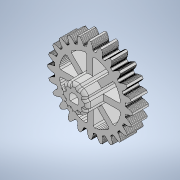
# Autodesk Inventor part: Ведущая шестерня дифференециала 24
Saved by Autodesk Inventor 2020 (Build 240168000, 168)
## iProperties
Created: 2021-10-09
Part Number: Ведущая шестерня дифференециала 24
Material: Типовые
Document SubType Name: Modeling
Designer: Антон
Density: 1 g/cm^3
Appearance: По умолчанию
Autodesk Inventor part; units mm, degrees
ref_plane "YZ Plane" through (0, 0, 0) normal (1, 0, 0) x (0, 1, 0)
ref_plane "XZ Plane" through (0, 0, 0) normal (0, 1, 0) x (-1, 0, 0)
ref_plane "XY Plane" through (0, 0, 0) normal (0, 0, 1) x (1, 0, 0)
sketch "a" plane through (0, 0, 0) normal (0, 0, 1) x (1, 0, 0)
  line L0 (2.2314, 12.0308) -> (2.1649, 12.1461)
  line L1 (2.1649, 12.1461) -> (2.1066, 12.1863)
  line L2 (2.1066, 12.1863) -> (2.0498, 12.2129)
  line L3 (2.0498, 12.2129) -> (1.9381, 12.246)
  line L4 (1.9381, 12.246) -> (1.8277, 12.2671)
  line L5 (1.8277, 12.2671) -> (1.7187, 12.2707)
  line L6 (1.7187, 12.2707) -> (1.4993, 12.2976)
  line L7 (1.4993, 12.2976) -> (1.2787, 12.3426)
  line L8 (1.2787, 12.3426) -> (1.0573, 12.4024)
  line L9 (1.0573, 12.4024) -> (0.8356, 12.4754)
  line L10 (0.8356, 12.4754) -> (0.6138, 12.5604)
  line L11 (0.6138, 12.5604) -> (0.3923, 12.6568)
  line L12 (0.3923, 12.6568) -> (0.1712, 12.7641)
  line L13 (0.1712, 12.7641) -> (0.0059, 12.8514)
  line L14 (0.0059, 12.8514) -> (0.0025, 13.5004)
  line L15 (0.0025, 13.5004) -> (0.1669, 13.5895)
  line L16 (0.1669, 13.5895) -> (0.3868, 13.699)
  line L17 (0.3868, 13.699) -> (0.6073, 13.7977)
  line L18 (0.6073, 13.7977) -> (0.8282, 13.8851)
  line L19 (0.8282, 13.8851) -> (1.0492, 13.9604)
  line L20 (1.0492, 13.9604) -> (1.2699, 14.0225)
  line L21 (1.2699, 14.0225) -> (1.49, 14.0699)
  line L22 (1.49, 14.0699) -> (1.7092, 14.099)
  line L23 (1.7092, 14.099) -> (1.818, 14.1038)
  line L24 (1.818, 14.1038) -> (1.9283, 14.126)
  line L25 (1.9283, 14.126) -> (2.0396, 14.1603)
  line L26 (2.0396, 14.1603) -> (2.0962, 14.1875)
  line L27 (2.0962, 14.1875) -> (2.154, 14.2283)
  line L28 (2.154, 14.2283) -> (2.2193, 14.3443)
  line L29 (2.2193, 14.3443) -> (2.2924, 14.9228)
  line L30 (2.2924, 14.9228) -> (2.258, 15.0513)
  line L31 (2.258, 15.0513) -> (2.2121, 15.1053)
  line L32 (2.2121, 15.1053) -> (2.1641, 15.1457)
  line L33 (2.1641, 15.1457) -> (2.0648, 15.2066)
  line L34 (2.0648, 15.2066) -> (1.9635, 15.2555)
  line L35 (1.9635, 15.2555) -> (1.8593, 15.2872)
  line L36 (1.8593, 15.2872) -> (1.6543, 15.3699)
  line L37 (1.6543, 15.3699) -> (1.4528, 15.4705)
  line L38 (1.4528, 15.4705) -> (1.2545, 15.5856)
  line L39 (1.2545, 15.5856) -> (1.0592, 15.7135)
  line L40 (1.0592, 15.7135) -> (0.867, 15.853)
  line L41 (0.867, 15.853) -> (0.6779, 16.0035)
  line L42 (0.6779, 16.0035) -> (0.4922, 16.1643)
  line L43 (0.4922, 16.1643) -> (0.355, 16.2914)
  line L44 (0.355, 16.2914) -> (0.5198, 16.9192)
  line L45 (0.5198, 16.9192) -> (0.7016, 16.9627)
  line L46 (0.7016, 16.9627) -> (0.9424, 17.0116)
  line L47 (0.9424, 17.0116) -> (1.181, 17.0498)
  line L48 (1.181, 17.0498) -> (1.4169, 17.077)
  line L49 (1.4169, 17.077) -> (1.6498, 17.0926)
  line L50 (1.6498, 17.0926) -> (1.8791, 17.0955)
  line L51 (1.8791, 17.0955) -> (2.104, 17.0842)
  line L52 (2.104, 17.0842) -> (2.3232, 17.0556)
  line L53 (2.3232, 17.0556) -> (2.4296, 17.0321)
  line L54 (2.4296, 17.0321) -> (2.5419, 17.025)
  line L55 (2.5419, 17.025) -> (2.6582, 17.0293)
  line L56 (2.6582, 17.0293) -> (2.7199, 17.041)
  line L57 (2.7199, 17.041) -> (2.7864, 17.0654)
  line L58 (2.7864, 17.0654) -> (2.8795, 17.1606)
  line L59 (2.8795, 17.1606) -> (3.0998, 17.7004)
  line L60 (3.0998, 17.7004) -> (3.0998, 17.8335)
  line L61 (3.0998, 17.8335) -> (3.0695, 17.8975)
  line L62 (3.0695, 17.8975) -> (3.0335, 17.9489)
  line L63 (3.0335, 17.9489) -> (2.9534, 18.0335)
  line L64 (2.9534, 18.0335) -> (2.8682, 18.1069)
  line L65 (2.8682, 18.1069) -> (2.7757, 18.1646)
  line L66 (2.7757, 18.1646) -> (2.5991, 18.2975)
  line L67 (2.5991, 18.2975) -> (2.4306, 18.4468)
  line L68 (2.4306, 18.4468) -> (2.2688, 18.6093)
  line L69 (2.2688, 18.6093) -> (2.1133, 18.7833)
  line L70 (2.1133, 18.7833) -> (1.9637, 18.9679)
  line L71 (1.9637, 18.9679) -> (1.82, 19.1621)
  line L72 (1.82, 19.1621) -> (1.6822, 19.3655)
  line L73 (1.6822, 19.3655) -> (1.5827, 19.5238)
  line L74 (1.5827, 19.5238) -> (1.9043, 20.0876)
  line L75 (1.9043, 20.0876) -> (2.0912, 20.0825)
  line L76 (2.0912, 20.0825) -> (2.3364, 20.0674)
  line L77 (2.3364, 20.0674) -> (2.5768, 20.0427)
  line L78 (2.5768, 20.0427) -> (2.8117, 20.0079)
  line L79 (2.8117, 20.0079) -> (3.0407, 19.9626)
  line L80 (3.0407, 19.9626) -> (3.2629, 19.9061)
  line L81 (3.2629, 19.9061) -> (3.4772, 19.837)
  line L82 (3.4772, 19.837) -> (3.6816, 19.7526)
  line L83 (3.6816, 19.7526) -> (3.7783, 19.7024)
  line L84 (3.7783, 19.7024) -> (3.8848, 19.6665)
  line L85 (3.8848, 19.6665) -> (3.9984, 19.6405)
  line L86 (3.9984, 19.6405) -> (4.061, 19.6358)
  line L87 (4.061, 19.6358) -> (4.1315, 19.6422)
  line L88 (4.1315, 19.6422) -> (4.246, 19.71)
  line L89 (4.246, 19.71) -> (4.5985, 20.1744)
  line L90 (4.5985, 20.1744) -> (4.633, 20.303)
  line L91 (4.633, 20.303) -> (4.6203, 20.3726)
  line L92 (4.6203, 20.3726) -> (4.5989, 20.4317)
  line L93 (4.5989, 20.4317) -> (4.5434, 20.534)
  line L94 (4.5434, 20.534) -> (4.4801, 20.627)
  line L95 (4.4801, 20.627) -> (4.4057, 20.7066)
  line L96 (4.4057, 20.7066) -> (4.2695, 20.8808)
  line L97 (4.2695, 20.8808) -> (4.1453, 21.0686)
  line L98 (4.1453, 21.0686) -> (4.0311, 21.2675)
  line L99 (4.0311, 21.2675) -> (3.9259, 21.4758)
  line L100 (3.9259, 21.4758) -> (3.8292, 21.6928)
  line L101 (3.8292, 21.6928) -> (3.7407, 21.9176)
  line L102 (3.7407, 21.9176) -> (3.6603, 22.1497)
  line L103 (3.6603, 22.1497) -> (3.6051, 22.3284)
  line L104 (3.6051, 22.3284) -> (4.0616, 22.7898)
  line L105 (4.0616, 22.7898) -> (4.2409, 22.7365)
  line L106 (4.2409, 22.7365) -> (4.4738, 22.6584)
  line L107 (4.4738, 22.6584) -> (4.6996, 22.5723)
  line L108 (4.6996, 22.5723) -> (4.9175, 22.4778)
  line L109 (4.9175, 22.4778) -> (5.127, 22.3748)
  line L110 (5.127, 22.3748) -> (5.327, 22.2627)
  line L111 (5.327, 22.2627) -> (5.5161, 22.1405)
  line L112 (5.5161, 22.1405) -> (5.6917, 22.0062)
  line L113 (5.6917, 22.0062) -> (5.7721, 21.9326)
  line L114 (5.7721, 21.9326) -> (5.8657, 21.8703)
  line L115 (5.8657, 21.8703) -> (5.9687, 21.8158)
  line L116 (5.9687, 21.8158) -> (6.0279, 21.7951)
  line L117 (6.0279, 21.7951) -> (6.0977, 21.783)
  line L118 (6.0977, 21.783) -> (6.2259, 21.8189)
  line L119 (6.2259, 21.8189) -> (6.6866, 22.1763)
  line L120 (6.6866, 22.1763) -> (6.7532, 22.2915)
  line L121 (6.7532, 22.2915) -> (6.7589, 22.3621)
  line L122 (6.7589, 22.3621) -> (6.7535, 22.4246)
  line L123 (6.7535, 22.4246) -> (6.7264, 22.5379)
  line L124 (6.7264, 22.5379) -> (6.6893, 22.6441)
  line L125 (6.6893, 22.6441) -> (6.638, 22.7402)
  line L126 (6.638, 22.7402) -> (6.5516, 22.9437)
  line L127 (6.5516, 22.9437) -> (6.4803, 23.1573)
  line L128 (6.4803, 23.1573) -> (6.4214, 23.3789)
  line L129 (6.4214, 23.3789) -> (6.3737, 23.6074)
  line L130 (6.3737, 23.6074) -> (6.3365, 23.842)
  line L131 (6.3365, 23.842) -> (6.3092, 24.082)
  line L132 (6.3092, 24.082) -> (6.2915, 24.3271)
  line L133 (6.2915, 24.3271) -> (6.2845, 24.5139)
  line L134 (6.2845, 24.5139) -> (6.8449, 24.8414)
  line L135 (6.8449, 24.8414) -> (7.0042, 24.7435)
  line L136 (7.0042, 24.7435) -> (7.209, 24.6078)
  line L137 (7.209, 24.6078) -> (7.4048, 24.4662)
  line L138 (7.4048, 24.4662) -> (7.5908, 24.3186)
  line L139 (7.5908, 24.3186) -> (7.7665, 24.1649)
  line L140 (7.7665, 24.1649) -> (7.9307, 24.0048)
  line L141 (7.9307, 24.0048) -> (8.0818, 23.8378)
  line L142 (8.0818, 23.8378) -> (8.2165, 23.6626)
  line L143 (8.2165, 23.6626) -> (8.2752, 23.5708)
  line L144 (8.2752, 23.5708) -> (8.3495, 23.4864)
  line L145 (8.3495, 23.4864) -> (8.4348, 23.4071)
  line L146 (8.4348, 23.4071) -> (8.4867, 23.3717)
  line L147 (8.4867, 23.3717) -> (8.551, 23.342)
  line L148 (8.551, 23.342) -> (8.6841, 23.3435)
  line L149 (8.6841, 23.3435) -> (9.2216, 23.5695)
  line L150 (9.2216, 23.5695) -> (9.3157, 23.6635)
  line L151 (9.3157, 23.6635) -> (9.3395, 23.7302)
  line L152 (9.3395, 23.7302) -> (9.3505, 23.792)
  line L153 (9.3505, 23.792) -> (9.3536, 23.9085)
  line L154 (9.3536, 23.9085) -> (9.3453, 24.0206)
  line L155 (9.3453, 24.0206) -> (9.3207, 24.1268)
  line L156 (9.3207, 24.1268) -> (9.2898, 24.3457)
  line L157 (9.2898, 24.3457) -> (9.2762, 24.5704)
  line L158 (9.2762, 24.5704) -> (9.2767, 24.7997)
  line L159 (9.2767, 24.7997) -> (9.2898, 25.0328)
  line L160 (9.2898, 25.0328) -> (9.3145, 25.269)
  line L161 (9.3145, 25.269) -> (9.3503, 25.508)
  line L162 (9.3503, 25.508) -> (9.3966, 25.7493)
  line L163 (9.3966, 25.7493) -> (9.4382, 25.9316)
  line L164 (9.4382, 25.9316) -> (10.0643, 26.1028)
  line L165 (10.0643, 26.1028) -> (10.1928, 25.9671)
  line L166 (10.1928, 25.9671) -> (10.3556, 25.783)
  line L167 (10.3556, 25.783) -> (10.508, 25.5955)
  line L168 (10.508, 25.5955) -> (10.6495, 25.4048)
  line L169 (10.6495, 25.4048) -> (10.7794, 25.2108)
  line L170 (10.7794, 25.2108) -> (10.8966, 25.0137)
  line L171 (10.8966, 25.0137) -> (10.9993, 24.8133)
  line L172 (10.9993, 24.8133) -> (11.0841, 24.6092)
  line L173 (11.0841, 24.6092) -> (11.117, 24.5053)
  line L174 (11.117, 24.5053) -> (11.1669, 24.4045)
  line L175 (11.1669, 24.4045) -> (11.2288, 24.3059)
  line L176 (11.2288, 24.3059) -> (11.2698, 24.2583)
  line L177 (11.2698, 24.2583) -> (11.3242, 24.213)
  line L178 (11.3242, 24.213) -> (11.4531, 24.1799)
  line L179 (11.4531, 24.1799) -> (12.0308, 24.2591)
  line L180 (12.0308, 24.2591) -> (12.1461, 24.3256)
  line L181 (12.1461, 24.3256) -> (12.1863, 24.3838)
  line L182 (12.1863, 24.3838) -> (12.2129, 24.4407)
  line L183 (12.2129, 24.4407) -> (12.246, 24.5523)
  line L184 (12.246, 24.5523) -> (12.2671, 24.6628)
  line L185 (12.2671, 24.6628) -> (12.2707, 24.7718)
  line L186 (12.2707, 24.7718) -> (12.2976, 24.9912)
  line L187 (12.2976, 24.9912) -> (12.3426, 25.2118)
  line L188 (12.3426, 25.2118) -> (12.4024, 25.4332)
  line L189 (12.4024, 25.4332) -> (12.4754, 25.6549)
  line L190 (12.4754, 25.6549) -> (12.5604, 25.8766)
  line L191 (12.5604, 25.8766) -> (12.6568, 26.0982)
  line L192 (12.6568, 26.0982) -> (12.7641, 26.3193)
  line L193 (12.7641, 26.3193) -> (12.8514, 26.4846)
  line L194 (12.8514, 26.4846) -> (13.5004, 26.488)
  line L195 (13.5004, 26.488) -> (13.5895, 26.3236)
  line L196 (13.5895, 26.3236) -> (13.699, 26.1036)
  line L197 (13.699, 26.1036) -> (13.7977, 25.8831)
  line L198 (13.7977, 25.8831) -> (13.8851, 25.6623)
  line L199 (13.8851, 25.6623) -> (13.9604, 25.4413)
  line L200 (13.9604, 25.4413) -> (14.0225, 25.2206)
  line L201 (14.0225, 25.2206) -> (14.0699, 25.0005)
  line L202 (14.0699, 25.0005) -> (14.099, 24.7813)
  line L203 (14.099, 24.7813) -> (14.1038, 24.6724)
  line L204 (14.1038, 24.6724) -> (14.126, 24.5622)
  line L205 (14.126, 24.5622) -> (14.1603, 24.4509)
  line L206 (14.1603, 24.4509) -> (14.1875, 24.3943)
  line L207 (14.1875, 24.3943) -> (14.2283, 24.3365)
  line L208 (14.2283, 24.3365) -> (14.3443, 24.2712)
  line L209 (14.3443, 24.2712) -> (14.9228, 24.1981)
  line L210 (14.9228, 24.1981) -> (15.0513, 24.2325)
  line L211 (15.0513, 24.2325) -> (15.1053, 24.2784)
  line L212 (15.1053, 24.2784) -> (15.1457, 24.3264)
  line L213 (15.1457, 24.3264) -> (15.2066, 24.4257)
  line L214 (15.2066, 24.4257) -> (15.2555, 24.5269)
  line L215 (15.2555, 24.5269) -> (15.2872, 24.6312)
  line L216 (15.2872, 24.6312) -> (15.3699, 24.8362)
  line L217 (15.3699, 24.8362) -> (15.4705, 25.0377)
  line L218 (15.4705, 25.0377) -> (15.5856, 25.236)
  line L219 (15.5856, 25.236) -> (15.7135, 25.4313)
  line L220 (15.7135, 25.4313) -> (15.853, 25.6235)
  line L221 (15.853, 25.6235) -> (16.0035, 25.8125)
  line L222 (16.0035, 25.8125) -> (16.1643, 25.9983)
  line L223 (16.1643, 25.9983) -> (16.2914, 26.1354)
  line L224 (16.2914, 26.1354) -> (16.9192, 25.9707)
  line L225 (16.9192, 25.9707) -> (16.9627, 25.7889)
  line L226 (16.9627, 25.7889) -> (17.0116, 25.5481)
  line L227 (17.0116, 25.5481) -> (17.0498, 25.3095)
  line L228 (17.0498, 25.3095) -> (17.077, 25.0736)
  line L229 (17.077, 25.0736) -> (17.0926, 24.8407)
  line L230 (17.0926, 24.8407) -> (17.0955, 24.6114)
  line L231 (17.0955, 24.6114) -> (17.0842, 24.3865)
  line L232 (17.0842, 24.3865) -> (17.0556, 24.1673)
  line L233 (17.0556, 24.1673) -> (17.0321, 24.0609)
  line L234 (17.0321, 24.0609) -> (17.025, 23.9486)
  line L235 (17.025, 23.9486) -> (17.0293, 23.8322)
  line L236 (17.0293, 23.8322) -> (17.041, 23.7705)
  line L237 (17.041, 23.7705) -> (17.0654, 23.7041)
  line L238 (17.0654, 23.7041) -> (17.1606, 23.611)
  line L239 (17.1606, 23.611) -> (17.7004, 23.3907)
  line L240 (17.7004, 23.3907) -> (17.8335, 23.3907)
  line L241 (17.8335, 23.3907) -> (17.8975, 23.421)
  line L242 (17.8975, 23.421) -> (17.9489, 23.4569)
  line L243 (17.9489, 23.4569) -> (18.0335, 23.5371)
  line L244 (18.0335, 23.5371) -> (18.1069, 23.6222)
  line L245 (18.1069, 23.6222) -> (18.1646, 23.7147)
  line L246 (18.1646, 23.7147) -> (18.2975, 23.8913)
  line L247 (18.2975, 23.8913) -> (18.4468, 24.0599)
  line L248 (18.4468, 24.0599) -> (18.6093, 24.2217)
  line L249 (18.6093, 24.2217) -> (18.7833, 24.3772)
  line L250 (18.7833, 24.3772) -> (18.9679, 24.5268)
  line L251 (18.9679, 24.5268) -> (19.1621, 24.6704)
  line L252 (19.1621, 24.6704) -> (19.3655, 24.8083)
  line L253 (19.3655, 24.8083) -> (19.5238, 24.9078)
  line L254 (19.5238, 24.9078) -> (20.0876, 24.5862)
  line L255 (20.0876, 24.5862) -> (20.0825, 24.3993)
  line L256 (20.0825, 24.3993) -> (20.0674, 24.1541)
  line L257 (20.0674, 24.1541) -> (20.0427, 23.9137)
  line L258 (20.0427, 23.9137) -> (20.0079, 23.6788)
  line L259 (20.0079, 23.6788) -> (19.9626, 23.4498)
  line L260 (19.9626, 23.4498) -> (19.9061, 23.2276)
  line L261 (19.9061, 23.2276) -> (19.837, 23.0132)
  line L262 (19.837, 23.0132) -> (19.7526, 22.8089)
  line L263 (19.7526, 22.8089) -> (19.7024, 22.7122)
  line L264 (19.7024, 22.7122) -> (19.6665, 22.6056)
  line L265 (19.6665, 22.6056) -> (19.6405, 22.4921)
  line L266 (19.6405, 22.4921) -> (19.6358, 22.4295)
  line L267 (19.6358, 22.4295) -> (19.6422, 22.359)
  line L268 (19.6422, 22.359) -> (19.71, 22.2445)
  line L269 (19.71, 22.2445) -> (20.1744, 21.8919)
  line L270 (20.1744, 21.8919) -> (20.303, 21.8574)
  line L271 (20.303, 21.8574) -> (20.3726, 21.8702)
  line L272 (20.3726, 21.8702) -> (20.4317, 21.8916)
  line L273 (20.4317, 21.8916) -> (20.534, 21.9471)
  line L274 (20.534, 21.9471) -> (20.627, 22.0104)
  line L275 (20.627, 22.0104) -> (20.7066, 22.0848)
  line L276 (20.7066, 22.0848) -> (20.8808, 22.221)
  line L277 (20.8808, 22.221) -> (21.0686, 22.3451)
  line L278 (21.0686, 22.3451) -> (21.2675, 22.4593)
  line L279 (21.2675, 22.4593) -> (21.4758, 22.5645)
  line L280 (21.4758, 22.5645) -> (21.6928, 22.6612)
  line L281 (21.6928, 22.6612) -> (21.9176, 22.7497)
  line L282 (21.9176, 22.7497) -> (22.1497, 22.8302)
  line L283 (22.1497, 22.8302) -> (22.3284, 22.8854)
  line L284 (22.3284, 22.8854) -> (22.7898, 22.4288)
  line L285 (22.7898, 22.4288) -> (22.7365, 22.2496)
  line L286 (22.7365, 22.2496) -> (22.6584, 22.0166)
  line L287 (22.6584, 22.0166) -> (22.5723, 21.7909)
  line L288 (22.5723, 21.7909) -> (22.4778, 21.5729)
  line L289 (22.4778, 21.5729) -> (22.3748, 21.3635)
  line L290 (22.3748, 21.3635) -> (22.2627, 21.1635)
  line L291 (22.2627, 21.1635) -> (22.1405, 20.9743)
  line L292 (22.1405, 20.9743) -> (22.0062, 20.7988)
  line L293 (22.0062, 20.7988) -> (21.9326, 20.7184)
  line L294 (21.9326, 20.7184) -> (21.8703, 20.6247)
  line L295 (21.8703, 20.6247) -> (21.8158, 20.5218)
  line L296 (21.8158, 20.5218) -> (21.7951, 20.4626)
  line L297 (21.7951, 20.4626) -> (21.783, 20.3928)
  line L298 (21.783, 20.3928) -> (21.8189, 20.2646)
  line L299 (21.8189, 20.2646) -> (22.1763, 19.8039)
  line L300 (22.1763, 19.8039) -> (22.2915, 19.7373)
  line L301 (22.2915, 19.7373) -> (22.3621, 19.7316)
  line L302 (22.3621, 19.7316) -> (22.4246, 19.737)
  line L303 (22.4246, 19.737) -> (22.5379, 19.7641)
  line L304 (22.5379, 19.7641) -> (22.6441, 19.8011)
  line L305 (22.6441, 19.8011) -> (22.7402, 19.8524)
  line L306 (22.7402, 19.8524) -> (22.9437, 19.9389)
  line L307 (22.9437, 19.9389) -> (23.1573, 20.0102)
  line L308 (23.1573, 20.0102) -> (23.3789, 20.0691)
  line L309 (23.3789, 20.0691) -> (23.6074, 20.1167)
  line L310 (23.6074, 20.1167) -> (23.842, 20.154)
  line L311 (23.842, 20.154) -> (24.082, 20.1813)
  line L312 (24.082, 20.1813) -> (24.3271, 20.199)
  line L313 (24.3271, 20.199) -> (24.5139, 20.206)
  line L314 (24.5139, 20.206) -> (24.8414, 19.6456)
  line L315 (24.8414, 19.6456) -> (24.7435, 19.4863)
  line L316 (24.7435, 19.4863) -> (24.6078, 19.2814)
  line L317 (24.6078, 19.2814) -> (24.4662, 19.0857)
  line L318 (24.4662, 19.0857) -> (24.3186, 18.8996)
  line L319 (24.3186, 18.8996) -> (24.1649, 18.724)
  line L320 (24.1649, 18.724) -> (24.0048, 18.5598)
  line L321 (24.0048, 18.5598) -> (23.8378, 18.4087)
  line L322 (23.8378, 18.4087) -> (23.6626, 18.2739)
  line L323 (23.6626, 18.2739) -> (23.5708, 18.2153)
  line L324 (23.5708, 18.2153) -> (23.4864, 18.141)
  line L325 (23.4864, 18.141) -> (23.4071, 18.0556)
  line L326 (23.4071, 18.0556) -> (23.3717, 18.0038)
  line L327 (23.3717, 18.0038) -> (23.342, 17.9395)
  line L328 (23.342, 17.9395) -> (23.3435, 17.8064)
  line L329 (23.3435, 17.8064) -> (23.5695, 17.2689)
  line L330 (23.5695, 17.2689) -> (23.6635, 17.1747)
  line L331 (23.6635, 17.1747) -> (23.7302, 17.151)
  line L332 (23.7302, 17.151) -> (23.792, 17.14)
  line L333 (23.792, 17.14) -> (23.9085, 17.1369)
  line L334 (23.9085, 17.1369) -> (24.0206, 17.1452)
  line L335 (24.0206, 17.1452) -> (24.1268, 17.1698)
  line L336 (24.1268, 17.1698) -> (24.3457, 17.2007)
  line L337 (24.3457, 17.2007) -> (24.5704, 17.2143)
  line L338 (24.5704, 17.2143) -> (24.7997, 17.2138)
  line L339 (24.7997, 17.2138) -> (25.0328, 17.2007)
  line L340 (25.0328, 17.2007) -> (25.269, 17.176)
  line L341 (25.269, 17.176) -> (25.508, 17.1402)
  line L342 (25.508, 17.1402) -> (25.7493, 17.0938)
  line L343 (25.7493, 17.0938) -> (25.9316, 17.0523)
  line L344 (25.9316, 17.0523) -> (26.1028, 16.4262)
  line L345 (26.1028, 16.4262) -> (25.9671, 16.2977)
  line L346 (25.9671, 16.2977) -> (25.783, 16.1349)
  line L347 (25.783, 16.1349) -> (25.5955, 15.9825)
  line L348 (25.5955, 15.9825) -> (25.4048, 15.8409)
  line L349 (25.4048, 15.8409) -> (25.2108, 15.7111)
  line L350 (25.2108, 15.7111) -> (25.0137, 15.5939)
  line L351 (25.0137, 15.5939) -> (24.8133, 15.4912)
  line L352 (24.8133, 15.4912) -> (24.6092, 15.4063)
  line L353 (24.6092, 15.4063) -> (24.5053, 15.3735)
  line L354 (24.5053, 15.3735) -> (24.4045, 15.3235)
  line L355 (24.4045, 15.3235) -> (24.3059, 15.2616)
  line L356 (24.3059, 15.2616) -> (24.2583, 15.2207)
  line L357 (24.2583, 15.2207) -> (24.213, 15.1663)
  line L358 (24.213, 15.1663) -> (24.1799, 15.0374)
  line L359 (24.1799, 15.0374) -> (24.2591, 14.4597)
  line L360 (24.2591, 14.4597) -> (24.3256, 14.3444)
  line L361 (24.3256, 14.3444) -> (24.3838, 14.3042)
  line L362 (24.3838, 14.3042) -> (24.4407, 14.2776)
  line L363 (24.4407, 14.2776) -> (24.5523, 14.2444)
  line L364 (24.5523, 14.2444) -> (24.6628, 14.2234)
  line L365 (24.6628, 14.2234) -> (24.7718, 14.2197)
  line L366 (24.7718, 14.2197) -> (24.9912, 14.1929)
  line L367 (24.9912, 14.1929) -> (25.2118, 14.1479)
  line L368 (25.2118, 14.1479) -> (25.4332, 14.088)
  line L369 (25.4332, 14.088) -> (25.6549, 14.0151)
  line L370 (25.6549, 14.0151) -> (25.8766, 13.9301)
  line L371 (25.8766, 13.9301) -> (26.0982, 13.8337)
  line L372 (26.0982, 13.8337) -> (26.3193, 13.7264)
  line L373 (26.3193, 13.7264) -> (26.4846, 13.6391)
  line L374 (26.4846, 13.6391) -> (26.488, 12.99)
  line L375 (26.488, 12.99) -> (26.3236, 12.901)
  line L376 (26.3236, 12.901) -> (26.1036, 12.7914)
  line L377 (26.1036, 12.7914) -> (25.8831, 12.6927)
  line L378 (25.8831, 12.6927) -> (25.6623, 12.6054)
  line L379 (25.6623, 12.6054) -> (25.4413, 12.5301)
  line L380 (25.4413, 12.5301) -> (25.2206, 12.468)
  line L381 (25.2206, 12.468) -> (25.0005, 12.4206)
  line L382 (25.0005, 12.4206) -> (24.7813, 12.3915)
  line L383 (24.7813, 12.3915) -> (24.6724, 12.3867)
  line L384 (24.6724, 12.3867) -> (24.5622, 12.3645)
  line L385 (24.5622, 12.3645) -> (24.4509, 12.3302)
  line L386 (24.4509, 12.3302) -> (24.3943, 12.303)
  line L387 (24.3943, 12.303) -> (24.3365, 12.2622)
  line L388 (24.3365, 12.2622) -> (24.2712, 12.1462)
  line L389 (24.2712, 12.1462) -> (24.1981, 11.5677)
  line L390 (24.1981, 11.5677) -> (24.2325, 11.4391)
  line L391 (24.2325, 11.4391) -> (24.2784, 11.3852)
  line L392 (24.2784, 11.3852) -> (24.3264, 11.3448)
  line L393 (24.3264, 11.3448) -> (24.4257, 11.2839)
  line L394 (24.4257, 11.2839) -> (24.5269, 11.235)
  line L395 (24.5269, 11.235) -> (24.6312, 11.2032)
  line L396 (24.6312, 11.2032) -> (24.8362, 11.1205)
  line L397 (24.8362, 11.1205) -> (25.0377, 11.0199)
  line L398 (25.0377, 11.0199) -> (25.236, 10.9048)
  line L399 (25.236, 10.9048) -> (25.4313, 10.777)
  line L400 (25.4313, 10.777) -> (25.6235, 10.6375)
  line L401 (25.6235, 10.6375) -> (25.8125, 10.487)
  line L402 (25.8125, 10.487) -> (25.9983, 10.3262)
  line L403 (25.9983, 10.3262) -> (26.1354, 10.1991)
  line L404 (26.1354, 10.1991) -> (25.9707, 9.5712)
  line L405 (25.9707, 9.5712) -> (25.7889, 9.5278)
  line L406 (25.7889, 9.5278) -> (25.5481, 9.4789)
  line L407 (25.5481, 9.4789) -> (25.3095, 9.4406)
  line L408 (25.3095, 9.4406) -> (25.0736, 9.4134)
  line L409 (25.0736, 9.4134) -> (24.8407, 9.3979)
  line L410 (24.8407, 9.3979) -> (24.6114, 9.395)
  line L411 (24.6114, 9.395) -> (24.3865, 9.4062)
  line L412 (24.3865, 9.4062) -> (24.1673, 9.4348)
  line L413 (24.1673, 9.4348) -> (24.0609, 9.4584)
  line L414 (24.0609, 9.4584) -> (23.9486, 9.4655)
  line L415 (23.9486, 9.4655) -> (23.8322, 9.4612)
  line L416 (23.8322, 9.4612) -> (23.7705, 9.4495)
  line L417 (23.7705, 9.4495) -> (23.7041, 9.4251)
  line L418 (23.7041, 9.4251) -> (23.611, 9.3299)
  line L419 (23.611, 9.3299) -> (23.3907, 8.7901)
  line L420 (23.3907, 8.7901) -> (23.3907, 8.657)
  line L421 (23.3907, 8.657) -> (23.421, 8.593)
  line L422 (23.421, 8.593) -> (23.4569, 8.5415)
  line L423 (23.4569, 8.5415) -> (23.5371, 8.457)
  line L424 (23.5371, 8.457) -> (23.6222, 8.3836)
  line L425 (23.6222, 8.3836) -> (23.7147, 8.3259)
  line L426 (23.7147, 8.3259) -> (23.8913, 8.193)
  line L427 (23.8913, 8.193) -> (24.0599, 8.0436)
  line L428 (24.0599, 8.0436) -> (24.2217, 7.8811)
  line L429 (24.2217, 7.8811) -> (24.3772, 7.7071)
  line L430 (24.3772, 7.7071) -> (24.5268, 7.5226)
  line L431 (24.5268, 7.5226) -> (24.6704, 7.3283)
  line L432 (24.6704, 7.3283) -> (24.8083, 7.1249)
  line L433 (24.8083, 7.1249) -> (24.9078, 6.9666)
  line L434 (24.9078, 6.9666) -> (24.5862, 6.4028)
  line L435 (24.5862, 6.4028) -> (24.3993, 6.4079)
  line L436 (24.3993, 6.4079) -> (24.1541, 6.423)
  line L437 (24.1541, 6.423) -> (23.9137, 6.4478)
  line L438 (23.9137, 6.4478) -> (23.6788, 6.4826)
  line L439 (23.6788, 6.4826) -> (23.4498, 6.5279)
  line L440 (23.4498, 6.5279) -> (23.2276, 6.5844)
  line L441 (23.2276, 6.5844) -> (23.0132, 6.6535)
  line L442 (23.0132, 6.6535) -> (22.8089, 6.7378)
  line L443 (22.8089, 6.7378) -> (22.7122, 6.7881)
  line L444 (22.7122, 6.7881) -> (22.6056, 6.824)
  line L445 (22.6056, 6.824) -> (22.4921, 6.85)
  line L446 (22.4921, 6.85) -> (22.4295, 6.8547)
  line L447 (22.4295, 6.8547) -> (22.359, 6.8483)
  line L448 (22.359, 6.8483) -> (22.2445, 6.7805)
  line L449 (22.2445, 6.7805) -> (21.8919, 6.316)
  line L450 (21.8919, 6.316) -> (21.8574, 6.1875)
  line L451 (21.8574, 6.1875) -> (21.8702, 6.1178)
  line L452 (21.8702, 6.1178) -> (21.8916, 6.0588)
  line L453 (21.8916, 6.0588) -> (21.9471, 5.9565)
  line L454 (21.9471, 5.9565) -> (22.0104, 5.8635)
  line L455 (22.0104, 5.8635) -> (22.0848, 5.7838)
  line L456 (22.0848, 5.7838) -> (22.221, 5.6097)
  line L457 (22.221, 5.6097) -> (22.3451, 5.4219)
  line L458 (22.3451, 5.4219) -> (22.4593, 5.223)
  line L459 (22.4593, 5.223) -> (22.5645, 5.0147)
  line L460 (22.5645, 5.0147) -> (22.6612, 4.7977)
  line L461 (22.6612, 4.7977) -> (22.7497, 4.5729)
  line L462 (22.7497, 4.5729) -> (22.8302, 4.3407)
  line L463 (22.8302, 4.3407) -> (22.8854, 4.1621)
  line L464 (22.8854, 4.1621) -> (22.4288, 3.7007)
  line L465 (22.4288, 3.7007) -> (22.2496, 3.754)
  line L466 (22.2496, 3.754) -> (22.0166, 3.8321)
  line L467 (22.0166, 3.8321) -> (21.7909, 3.9182)
  line L468 (21.7909, 3.9182) -> (21.5729, 4.0126)
  line L469 (21.5729, 4.0126) -> (21.3635, 4.1156)
  line L470 (21.3635, 4.1156) -> (21.1635, 4.2278)
  line L471 (21.1635, 4.2278) -> (20.9743, 4.3499)
  line L472 (20.9743, 4.3499) -> (20.7988, 4.4843)
  line L473 (20.7988, 4.4843) -> (20.7184, 4.5579)
  line L474 (20.7184, 4.5579) -> (20.6247, 4.6202)
  line L475 (20.6247, 4.6202) -> (20.5218, 4.6746)
  line L476 (20.5218, 4.6746) -> (20.4626, 4.6954)
  line L477 (20.4626, 4.6954) -> (20.3928, 4.7074)
  line L478 (20.3928, 4.7074) -> (20.2646, 4.6716)
  line L479 (20.2646, 4.6716) -> (19.8039, 4.3142)
  line L480 (19.8039, 4.3142) -> (19.7373, 4.199)
  line L481 (19.7373, 4.199) -> (19.7316, 4.1284)
  line L482 (19.7316, 4.1284) -> (19.737, 4.0659)
  line L483 (19.737, 4.0659) -> (19.7641, 3.9526)
  line L484 (19.7641, 3.9526) -> (19.8011, 3.8464)
  line L485 (19.8011, 3.8464) -> (19.8524, 3.7502)
  line L486 (19.8524, 3.7502) -> (19.9389, 3.5468)
  line L487 (19.9389, 3.5468) -> (20.0102, 3.3332)
  line L488 (20.0102, 3.3332) -> (20.0691, 3.1116)
  line L489 (20.0691, 3.1116) -> (20.1167, 2.8831)
  line L490 (20.1167, 2.8831) -> (20.154, 2.6485)
  line L491 (20.154, 2.6485) -> (20.1813, 2.4085)
  line L492 (20.1813, 2.4085) -> (20.199, 2.1634)
  line L493 (20.199, 2.1634) -> (20.206, 1.9765)
  line L494 (20.206, 1.9765) -> (19.6456, 1.649)
  line L495 (19.6456, 1.649) -> (19.4863, 1.7469)
  line L496 (19.4863, 1.7469) -> (19.2814, 1.8826)
  line L497 (19.2814, 1.8826) -> (19.0857, 2.0242)
  line L498 (19.0857, 2.0242) -> (18.8996, 2.1719)
  line L499 (18.8996, 2.1719) -> (18.724, 2.3256)
  line L500 (18.724, 2.3256) -> (18.5598, 2.4856)
  line L501 (18.5598, 2.4856) -> (18.4087, 2.6526)
  line L502 (18.4087, 2.6526) -> (18.2739, 2.8278)
  line L503 (18.2739, 2.8278) -> (18.2153, 2.9197)
  line L504 (18.2153, 2.9197) -> (18.141, 3.0041)
  line L505 (18.141, 3.0041) -> (18.0556, 3.0834)
  line L506 (18.0556, 3.0834) -> (18.0038, 3.1187)
  line L507 (18.0038, 3.1187) -> (17.9395, 3.1484)
  line L508 (17.9395, 3.1484) -> (17.8064, 3.147)
  line L509 (17.8064, 3.147) -> (17.2689, 2.921)
  line L510 (17.2689, 2.921) -> (17.1747, 2.827)
  line L511 (17.1747, 2.827) -> (17.151, 2.7603)
  line L512 (17.151, 2.7603) -> (17.14, 2.6985)
  line L513 (17.14, 2.6985) -> (17.1369, 2.582)
  line L514 (17.1369, 2.582) -> (17.1452, 2.4699)
  line L515 (17.1452, 2.4699) -> (17.1698, 2.3637)
  line L516 (17.1698, 2.3637) -> (17.2007, 2.1448)
  line L517 (17.2007, 2.1448) -> (17.2143, 1.92)
  line L518 (17.2143, 1.92) -> (17.2138, 1.6907)
  line L519 (17.2138, 1.6907) -> (17.2007, 1.4577)
  line L520 (17.2007, 1.4577) -> (17.176, 1.2215)
  line L521 (17.176, 1.2215) -> (17.1402, 0.9825)
  line L522 (17.1402, 0.9825) -> (17.0938, 0.7412)
  line L523 (17.0938, 0.7412) -> (17.0523, 0.5589)
  line L524 (17.0523, 0.5589) -> (16.4262, 0.3876)
  line L525 (16.4262, 0.3876) -> (16.2977, 0.5234)
  line L526 (16.2977, 0.5234) -> (16.1349, 0.7075)
  line L527 (16.1349, 0.7075) -> (15.9825, 0.895)
  line L528 (15.9825, 0.895) -> (15.8409, 1.0857)
  line L529 (15.8409, 1.0857) -> (15.7111, 1.2796)
  line L530 (15.7111, 1.2796) -> (15.5939, 1.4768)
  line L531 (15.5939, 1.4768) -> (15.4912, 1.6772)
  line L532 (15.4912, 1.6772) -> (15.4063, 1.8813)
  line L533 (15.4063, 1.8813) -> (15.3735, 1.9852)
  line L534 (15.3735, 1.9852) -> (15.3235, 2.0859)
  line L535 (15.3235, 2.0859) -> (15.2616, 2.1846)
  line L536 (15.2616, 2.1846) -> (15.2207, 2.2322)
  line L537 (15.2207, 2.2322) -> (15.1663, 2.2775)
  line L538 (15.1663, 2.2775) -> (15.0374, 2.3105)
  line L539 (15.0374, 2.3105) -> (14.4597, 2.2314)
  line L540 (14.4597, 2.2314) -> (14.3444, 2.1649)
  line L541 (14.3444, 2.1649) -> (14.3042, 2.1066)
  line L542 (14.3042, 2.1066) -> (14.2776, 2.0498)
  line L543 (14.2776, 2.0498) -> (14.2444, 1.9381)
  line L544 (14.2444, 1.9381) -> (14.2234, 1.8277)
  line L545 (14.2234, 1.8277) -> (14.2197, 1.7187)
  line L546 (14.2197, 1.7187) -> (14.1929, 1.4993)
  line L547 (14.1929, 1.4993) -> (14.1479, 1.2787)
  line L548 (14.1479, 1.2787) -> (14.088, 1.0573)
  line L549 (14.088, 1.0573) -> (14.0151, 0.8356)
  line L550 (14.0151, 0.8356) -> (13.9301, 0.6138)
  line L551 (13.9301, 0.6138) -> (13.8337, 0.3923)
  line L552 (13.8337, 0.3923) -> (13.7264, 0.1712)
  line L553 (13.7264, 0.1712) -> (13.6391, 0.0059)
  line L554 (13.6391, 0.0059) -> (12.99, 0.0025)
  line L555 (12.99, 0.0025) -> (12.901, 0.1669)
  line L556 (12.901, 0.1669) -> (12.7914, 0.3868)
  line L557 (12.7914, 0.3868) -> (12.6927, 0.6073)
  line L558 (12.6927, 0.6073) -> (12.6054, 0.8282)
  line L559 (12.6054, 0.8282) -> (12.5301, 1.0492)
  line L560 (12.5301, 1.0492) -> (12.468, 1.2699)
  line L561 (12.468, 1.2699) -> (12.4206, 1.49)
  line L562 (12.4206, 1.49) -> (12.3915, 1.7092)
  line L563 (12.3915, 1.7092) -> (12.3867, 1.818)
  line L564 (12.3867, 1.818) -> (12.3645, 1.9283)
  line L565 (12.3645, 1.9283) -> (12.3302, 2.0396)
  line L566 (12.3302, 2.0396) -> (12.303, 2.0962)
  line L567 (12.303, 2.0962) -> (12.2622, 2.154)
  line L568 (12.2622, 2.154) -> (12.1462, 2.2193)
  line L569 (12.1462, 2.2193) -> (11.5677, 2.2924)
  line L570 (11.5677, 2.2924) -> (11.4391, 2.258)
  line L571 (11.4391, 2.258) -> (11.3852, 2.2121)
  line L572 (11.3852, 2.2121) -> (11.3448, 2.1641)
  line L573 (11.3448, 2.1641) -> (11.2839, 2.0648)
  line L574 (11.2839, 2.0648) -> (11.235, 1.9635)
  line L575 (11.235, 1.9635) -> (11.2032, 1.8593)
  line L576 (11.2032, 1.8593) -> (11.1205, 1.6543)
  line L577 (11.1205, 1.6543) -> (11.0199, 1.4528)
  line L578 (11.0199, 1.4528) -> (10.9048, 1.2545)
  line L579 (10.9048, 1.2545) -> (10.777, 1.0592)
  line L580 (10.777, 1.0592) -> (10.6375, 0.867)
  line L581 (10.6375, 0.867) -> (10.487, 0.6779)
  line L582 (10.487, 0.6779) -> (10.3262, 0.4922)
  line L583 (10.3262, 0.4922) -> (10.1991, 0.355)
  line L584 (10.1991, 0.355) -> (9.5712, 0.5198)
  line L585 (9.5712, 0.5198) -> (9.5278, 0.7016)
  line L586 (9.5278, 0.7016) -> (9.4789, 0.9424)
  line L587 (9.4789, 0.9424) -> (9.4406, 1.181)
  line L588 (9.4406, 1.181) -> (9.4134, 1.4169)
  line L589 (9.4134, 1.4169) -> (9.3979, 1.6498)
  line L590 (9.3979, 1.6498) -> (9.395, 1.8791)
  line L591 (9.395, 1.8791) -> (9.4062, 2.104)
  line L592 (9.4062, 2.104) -> (9.4348, 2.3232)
  line L593 (9.4348, 2.3232) -> (9.4584, 2.4296)
  line L594 (9.4584, 2.4296) -> (9.4655, 2.5419)
  line L595 (9.4655, 2.5419) -> (9.4612, 2.6582)
  line L596 (9.4612, 2.6582) -> (9.4495, 2.7199)
  line L597 (9.4495, 2.7199) -> (9.4251, 2.7864)
  line L598 (9.4251, 2.7864) -> (9.3299, 2.8795)
  line L599 (9.3299, 2.8795) -> (8.7901, 3.0998)
  line L600 (8.7901, 3.0998) -> (8.657, 3.0998)
  line L601 (8.657, 3.0998) -> (8.593, 3.0695)
  line L602 (8.593, 3.0695) -> (8.5415, 3.0335)
  line L603 (8.5415, 3.0335) -> (8.457, 2.9534)
  line L604 (8.457, 2.9534) -> (8.3836, 2.8682)
  line L605 (8.3836, 2.8682) -> (8.3259, 2.7757)
  line L606 (8.3259, 2.7757) -> (8.193, 2.5991)
  line L607 (8.193, 2.5991) -> (8.0436, 2.4306)
  line L608 (8.0436, 2.4306) -> (7.8811, 2.2688)
  line L609 (7.8811, 2.2688) -> (7.7071, 2.1133)
  line L610 (7.7071, 2.1133) -> (7.5226, 1.9637)
  line L611 (7.5226, 1.9637) -> (7.3283, 1.82)
  line L612 (7.3283, 1.82) -> (7.1249, 1.6822)
  line L613 (7.1249, 1.6822) -> (6.9666, 1.5827)
  line L614 (6.9666, 1.5827) -> (6.4028, 1.9043)
  line L615 (6.4028, 1.9043) -> (6.4079, 2.0912)
  line L616 (6.4079, 2.0912) -> (6.423, 2.3364)
  line L617 (6.423, 2.3364) -> (6.4478, 2.5768)
  line L618 (6.4478, 2.5768) -> (6.4826, 2.8117)
  line L619 (6.4826, 2.8117) -> (6.5279, 3.0407)
  line L620 (6.5279, 3.0407) -> (6.5844, 3.2629)
  line L621 (6.5844, 3.2629) -> (6.6535, 3.4772)
  line L622 (6.6535, 3.4772) -> (6.7378, 3.6816)
  line L623 (6.7378, 3.6816) -> (6.7881, 3.7783)
  line L624 (6.7881, 3.7783) -> (6.824, 3.8848)
  line L625 (6.824, 3.8848) -> (6.85, 3.9984)
  line L626 (6.85, 3.9984) -> (6.8547, 4.061)
  line L627 (6.8547, 4.061) -> (6.8483, 4.1315)
  line L628 (6.8483, 4.1315) -> (6.7805, 4.246)
  line L629 (6.7805, 4.246) -> (6.316, 4.5985)
  line L630 (6.316, 4.5985) -> (6.1875, 4.633)
  line L631 (6.1875, 4.633) -> (6.1178, 4.6203)
  line L632 (6.1178, 4.6203) -> (6.0588, 4.5989)
  line L633 (6.0588, 4.5989) -> (5.9565, 4.5434)
  line L634 (5.9565, 4.5434) -> (5.8635, 4.4801)
  line L635 (5.8635, 4.4801) -> (5.7838, 4.4057)
  line L636 (5.7838, 4.4057) -> (5.6097, 4.2695)
  line L637 (5.6097, 4.2695) -> (5.4219, 4.1453)
  line L638 (5.4219, 4.1453) -> (5.223, 4.0311)
  line L639 (5.223, 4.0311) -> (5.0147, 3.9259)
  line L640 (5.0147, 3.9259) -> (4.7977, 3.8292)
  line L641 (4.7977, 3.8292) -> (4.5729, 3.7407)
  line L642 (4.5729, 3.7407) -> (4.3407, 3.6603)
  line L643 (4.3407, 3.6603) -> (4.1621, 3.6051)
  line L644 (4.1621, 3.6051) -> (3.7007, 4.0616)
  line L645 (3.7007, 4.0616) -> (3.754, 4.2409)
  line L646 (3.754, 4.2409) -> (3.8321, 4.4738)
  line L647 (3.8321, 4.4738) -> (3.9182, 4.6996)
  line L648 (3.9182, 4.6996) -> (4.0126, 4.9175)
  line L649 (4.0126, 4.9175) -> (4.1156, 5.127)
  line L650 (4.1156, 5.127) -> (4.2278, 5.327)
  line L651 (4.2278, 5.327) -> (4.3499, 5.5161)
  line L652 (4.3499, 5.5161) -> (4.4843, 5.6917)
  line L653 (4.4843, 5.6917) -> (4.5579, 5.7721)
  line L654 (4.5579, 5.7721) -> (4.6202, 5.8657)
  line L655 (4.6202, 5.8657) -> (4.6746, 5.9687)
  line L656 (4.6746, 5.9687) -> (4.6954, 6.0279)
  line L657 (4.6954, 6.0279) -> (4.7074, 6.0977)
  line L658 (4.7074, 6.0977) -> (4.6716, 6.2259)
  line L659 (4.6716, 6.2259) -> (4.3142, 6.6866)
  line L660 (4.3142, 6.6866) -> (4.199, 6.7532)
  line L661 (4.199, 6.7532) -> (4.1284, 6.7589)
  line L662 (4.1284, 6.7589) -> (4.0659, 6.7535)
  line L663 (4.0659, 6.7535) -> (3.9526, 6.7264)
  line L664 (3.9526, 6.7264) -> (3.8464, 6.6893)
  line L665 (3.8464, 6.6893) -> (3.7502, 6.638)
  line L666 (3.7502, 6.638) -> (3.5468, 6.5516)
  line L667 (3.5468, 6.5516) -> (3.3332, 6.4803)
  line L668 (3.3332, 6.4803) -> (3.1116, 6.4214)
  line L669 (3.1116, 6.4214) -> (2.8831, 6.3737)
  line L670 (2.8831, 6.3737) -> (2.6485, 6.3365)
  line L671 (2.6485, 6.3365) -> (2.4085, 6.3092)
  line L672 (2.4085, 6.3092) -> (2.1634, 6.2915)
  line L673 (2.1634, 6.2915) -> (1.9765, 6.2845)
  line L674 (1.9765, 6.2845) -> (1.649, 6.8449)
  line L675 (1.649, 6.8449) -> (1.7469, 7.0042)
  line L676 (1.7469, 7.0042) -> (1.8826, 7.209)
  line L677 (1.8826, 7.209) -> (2.0242, 7.4048)
  line L678 (2.0242, 7.4048) -> (2.1719, 7.5908)
  line L679 (2.1719, 7.5908) -> (2.3256, 7.7665)
  line L680 (2.3256, 7.7665) -> (2.4856, 7.9307)
  line L681 (2.4856, 7.9307) -> (2.6526, 8.0818)
  line L682 (2.6526, 8.0818) -> (2.8278, 8.2165)
  line L683 (2.8278, 8.2165) -> (2.9197, 8.2752)
  line L684 (2.9197, 8.2752) -> (3.0041, 8.3495)
  line L685 (3.0041, 8.3495) -> (3.0834, 8.4348)
  line L686 (3.0834, 8.4348) -> (3.1187, 8.4867)
  line L687 (3.1187, 8.4867) -> (3.1484, 8.551)
  line L688 (3.1484, 8.551) -> (3.147, 8.6841)
  line L689 (3.147, 8.6841) -> (2.921, 9.2216)
  line L690 (2.921, 9.2216) -> (2.827, 9.3157)
  line L691 (2.827, 9.3157) -> (2.7603, 9.3395)
  line L692 (2.7603, 9.3395) -> (2.6985, 9.3505)
  line L693 (2.6985, 9.3505) -> (2.582, 9.3536)
  line L694 (2.582, 9.3536) -> (2.4699, 9.3453)
  line L695 (2.4699, 9.3453) -> (2.3637, 9.3207)
  line L696 (2.3637, 9.3207) -> (2.1448, 9.2898)
  line L697 (2.1448, 9.2898) -> (1.92, 9.2762)
  line L698 (1.92, 9.2762) -> (1.6907, 9.2767)
  line L699 (1.6907, 9.2767) -> (1.4577, 9.2898)
  line L700 (1.4577, 9.2898) -> (1.2215, 9.3145)
  line L701 (1.2215, 9.3145) -> (0.9825, 9.3503)
  line L702 (0.9825, 9.3503) -> (0.7412, 9.3966)
  line L703 (0.7412, 9.3966) -> (0.5589, 9.4382)
  line L704 (0.5589, 9.4382) -> (0.3876, 10.0643)
  line L705 (0.3876, 10.0643) -> (0.5234, 10.1928)
  line L706 (0.5234, 10.1928) -> (0.7075, 10.3556)
  line L707 (0.7075, 10.3556) -> (0.895, 10.508)
  line L708 (0.895, 10.508) -> (1.0857, 10.6495)
  line L709 (1.0857, 10.6495) -> (1.2796, 10.7794)
  line L710 (1.2796, 10.7794) -> (1.4768, 10.8966)
  line L711 (1.4768, 10.8966) -> (1.6772, 10.9993)
  line L712 (1.6772, 10.9993) -> (1.8813, 11.0841)
  line L713 (1.8813, 11.0841) -> (1.9852, 11.117)
  line L714 (1.9852, 11.117) -> (2.0859, 11.1669)
  line L715 (2.0859, 11.1669) -> (2.1846, 11.2288)
  line L716 (2.1846, 11.2288) -> (2.2322, 11.2698)
  line L717 (2.2322, 11.2698) -> (2.2775, 11.3242)
  line L718 (2.2775, 11.3242) -> (2.3105, 11.4531)
  line L719 (2.3105, 11.4531) -> (2.2314, 12.0308)
  line L720 (9.1522, 12.2685) -> (4.1277, 12.2422)
  line L721 (4.1277, 12.2422) -> (3.7122, 11.7624)
  line L722 (3.7122, 11.7624) -> (3.8384, 11.1029)
  line L723 (3.8384, 11.1029) -> (4.0102, 10.4539)
  line L724 (4.0102, 10.4539) -> (4.2267, 9.8184)
  line L725 (4.2267, 9.8184) -> (4.4869, 9.1994)
  line L726 (4.4869, 9.1994) -> (4.7895, 8.6)
  line L727 (4.7895, 8.6) -> (5.133, 8.0232)
  line L728 (5.133, 8.0232) -> (5.5159, 7.4716)
  line L729 (5.5159, 7.4716) -> (6.1494, 7.4328)
  line L730 (6.1494, 7.4328) -> (9.6836, 11.0042)
  line L731 (9.6836, 11.0042) -> (9.7934, 11.7942)
  line L732 (9.7934, 11.7942) -> (9.1522, 12.2685)
  line L733 (11.0417, 9.6604) -> (7.5074, 6.0889)
  line L734 (7.5074, 6.0889) -> (7.5529, 5.4558)
  line L735 (7.5529, 5.4558) -> (8.1084, 5.0788)
  line L736 (8.1084, 5.0788) -> (8.6889, 4.7413)
  line L737 (8.6889, 4.7413) -> (9.2913, 4.445)
  line L738 (9.2913, 4.445) -> (9.913, 4.1913)
  line L739 (9.913, 4.1913) -> (10.5508, 3.9815)
  line L740 (10.5508, 3.9815) -> (11.2016, 3.8165)
  line L741 (11.2016, 3.8165) -> (11.8623, 3.6972)
  line L742 (11.8623, 3.6972) -> (12.3377, 4.1177)
  line L743 (12.3377, 4.1177) -> (12.3114, 9.1422)
  line L744 (12.3114, 9.1422) -> (11.8305, 9.7784)
  line L745 (11.8305, 9.7784) -> (11.0417, 9.6604)
  line L746 (14.222, 9.1522) -> (14.2483, 4.1277)
  line L747 (14.2483, 4.1277) -> (14.7281, 3.7122)
  line L748 (14.7281, 3.7122) -> (15.3875, 3.8384)
  line L749 (15.3875, 3.8384) -> (16.0366, 4.0102)
  line L750 (16.0366, 4.0102) -> (16.6721, 4.2267)
  line L751 (16.6721, 4.2267) -> (17.2911, 4.4869)
  line L752 (17.2911, 4.4869) -> (17.8904, 4.7895)
  line L753 (17.8904, 4.7895) -> (18.4673, 5.133)
  line L754 (18.4673, 5.133) -> (19.0188, 5.5159)
  line L755 (19.0188, 5.5159) -> (19.0577, 6.1494)
  line L756 (19.0577, 6.1494) -> (15.4862, 9.6836)
  line L757 (15.4862, 9.6836) -> (14.6962, 9.7934)
  line L758 (14.6962, 9.7934) -> (14.222, 9.1522)
  line L759 (16.8301, 11.0417) -> (20.4015, 7.5074)
  line L760 (20.4015, 7.5074) -> (21.0346, 7.5529)
  line L761 (21.0346, 7.5529) -> (21.4117, 8.1084)
  line L762 (21.4117, 8.1084) -> (21.7492, 8.6889)
  line L763 (21.7492, 8.6889) -> (22.0455, 9.2913)
  line L764 (22.0455, 9.2913) -> (22.2992, 9.913)
  line L765 (22.2992, 9.913) -> (22.509, 10.5508)
  line L766 (22.509, 10.5508) -> (22.674, 11.2016)
  line L767 (22.674, 11.2016) -> (22.7933, 11.8623)
  line L768 (22.7933, 11.8623) -> (22.3727, 12.3377)
  line L769 (22.3727, 12.3377) -> (17.3483, 12.3114)
  line L770 (17.3483, 12.3114) -> (16.712, 11.8305)
  line L771 (16.712, 11.8305) -> (16.8301, 11.0417)
  line L772 (17.3383, 14.222) -> (22.3627, 14.2483)
  line L773 (22.3627, 14.2483) -> (22.7783, 14.7281)
  line L774 (22.7783, 14.7281) -> (22.6521, 15.3875)
  line L775 (22.6521, 15.3875) -> (22.4803, 16.0366)
  line L776 (22.4803, 16.0366) -> (22.2638, 16.6721)
  line L777 (22.2638, 16.6721) -> (22.0036, 17.2911)
  line L778 (22.0036, 17.2911) -> (21.701, 17.8904)
  line L779 (21.701, 17.8904) -> (21.3575, 18.4673)
  line L780 (21.3575, 18.4673) -> (20.9746, 19.0188)
  line L781 (20.9746, 19.0188) -> (20.341, 19.0577)
  line L782 (20.341, 19.0577) -> (16.8068, 15.4862)
  line L783 (16.8068, 15.4862) -> (16.697, 14.6962)
  line L784 (16.697, 14.6962) -> (17.3383, 14.222)
  line L785 (15.4488, 16.8301) -> (18.983, 20.4015)
  line L786 (18.983, 20.4015) -> (18.9376, 21.0346)
  line L787 (18.9376, 21.0346) -> (18.382, 21.4117)
  line L788 (18.382, 21.4117) -> (17.8016, 21.7492)
  line L789 (17.8016, 21.7492) -> (17.1991, 22.0455)
  line L790 (17.1991, 22.0455) -> (16.5775, 22.2992)
  line L791 (16.5775, 22.2992) -> (15.9397, 22.509)
  line L792 (15.9397, 22.509) -> (15.2889, 22.674)
  line L793 (15.2889, 22.674) -> (14.6282, 22.7933)
  line L794 (14.6282, 22.7933) -> (14.1527, 22.3727)
  line L795 (14.1527, 22.3727) -> (14.179, 17.3483)
  line L796 (14.179, 17.3483) -> (14.66, 16.712)
  line L797 (14.66, 16.712) -> (15.4488, 16.8301)
  line L798 (12.2685, 17.3383) -> (12.2422, 22.3627)
  line L799 (12.2422, 22.3627) -> (11.7624, 22.7783)
  line L800 (11.7624, 22.7783) -> (11.1029, 22.6521)
  line L801 (11.1029, 22.6521) -> (10.4539, 22.4803)
  line L802 (10.4539, 22.4803) -> (9.8184, 22.2638)
  line L803 (9.8184, 22.2638) -> (9.1994, 22.0036)
  line L804 (9.1994, 22.0036) -> (8.6, 21.701)
  line L805 (8.6, 21.701) -> (8.0232, 21.3575)
  line L806 (8.0232, 21.3575) -> (7.4716, 20.9746)
  line L807 (7.4716, 20.9746) -> (7.4328, 20.341)
  line L808 (7.4328, 20.341) -> (11.0042, 16.8068)
  line L809 (11.0042, 16.8068) -> (11.7942, 16.697)
  line L810 (11.7942, 16.697) -> (12.2685, 17.3383)
  line L811 (9.6604, 15.4488) -> (6.0889, 18.983)
  line L812 (6.0889, 18.983) -> (5.4558, 18.9376)
  line L813 (5.4558, 18.9376) -> (5.0788, 18.382)
  line L814 (5.0788, 18.382) -> (4.7413, 17.8016)
  line L815 (4.7413, 17.8016) -> (4.445, 17.1991)
  line L816 (4.445, 17.1991) -> (4.1913, 16.5775)
  line L817 (4.1913, 16.5775) -> (3.9815, 15.9397)
  line L818 (3.9815, 15.9397) -> (3.8165, 15.2889)
  line L819 (3.8165, 15.2889) -> (3.6972, 14.6282)
  line L820 (3.6972, 14.6282) -> (4.1177, 14.1527)
  line L821 (4.1177, 14.1527) -> (9.1422, 14.179)
  line L822 (9.1422, 14.179) -> (9.7784, 14.66)
  line L823 (9.7784, 14.66) -> (9.6604, 15.4488)
  circle A0 centre (13.2452, 13.2452) radius 1.5
  constraints: 1648 end point, 1 centre point
extrude "Выдавливание1" add sketch "a" along normal blind 5
sketch "Эскиз3" plane through (0, 0, 5) normal (0, 0, 1) x (1, 0, 0)
  circle A0 centre (13.2452, 13.2452) radius 1.5 projected
  line L0 (12.2685, 17.3383) -> (11.7942, 16.697) projected
  circle A1 centre (13.2452, 13.2452) radius 4.208
  line L1 (11.7942, 16.697) -> (11.0042, 16.8068) projected
  line L2 (11.7942, 16.697) -> (11.0042, 16.8068)
  line L3 (11.7942, 16.697) -> (12.2685, 17.3383)
  line L4 (14.66, 16.712) -> (14.179, 17.3483) projected
  line L5 (14.179, 17.3483) -> (14.66, 16.712)
  line L6 (15.4488, 16.8301) -> (14.66, 16.712) projected
  line L7 (14.66, 16.712) -> (15.4488, 16.8301)
  line L8 (16.697, 14.6962) -> (16.8068, 15.4862) projected
  line L9 (17.3383, 14.222) -> (16.697, 14.6962) projected
  line L10 (16.8068, 15.4862) -> (16.697, 14.6962)
  line L11 (16.697, 14.6962) -> (17.3383, 14.222)
  line L12 (16.712, 11.8305) -> (17.3483, 12.3114) projected
  line L13 (16.712, 11.8305) -> (17.3483, 12.3114)
  line L14 (16.8301, 11.0417) -> (16.712, 11.8305) projected
  line L15 (16.712, 11.8305) -> (16.8301, 11.0417)
  line L16 (15.4862, 9.6836) -> (19.0577, 6.1494) projected
  line L17 (14.6962, 9.7934) -> (15.4862, 9.6836) projected
  line L18 (15.4862, 9.6836) -> (14.6962, 9.7934)
  line L19 (14.222, 9.1522) -> (14.6962, 9.7934) projected
  line L20 (14.2483, 4.1277) -> (14.222, 9.1522) projected
  line L21 (14.6962, 9.7934) -> (14.222, 9.1522)
  line L22 (7.5074, 6.0889) -> (11.0417, 9.6604) projected
  line L23 (11.8305, 9.7784) -> (12.3114, 9.1422) projected
  line L24 (11.0417, 9.6604) -> (11.8305, 9.7784)
  line L25 (11.0417, 9.6604) -> (11.8305, 9.7784) projected
  line L26 (11.8305, 9.7784) -> (12.3114, 9.1422)
  line L27 (9.6836, 11.0042) -> (6.1494, 7.4328) projected
  line L28 (9.7934, 11.7942) -> (9.6836, 11.0042) projected
  line L29 (9.6836, 11.0042) -> (9.7934, 11.7942)
  line L30 (4.1277, 12.2422) -> (9.1522, 12.2685) projected
  line L31 (9.7934, 11.7942) -> (9.1522, 12.2685)
  line L32 (9.7784, 14.66) -> (9.1422, 14.179) projected
  line L33 (9.1422, 14.179) -> (9.7784, 14.66)
  line L34 (9.7784, 14.66) -> (9.6604, 15.4488)
  line L35 (9.6604, 15.4488) -> (9.7784, 14.66) projected
  circle A2 centre (13.2452, 13.2452) radius 1.5
  point P0 (0, 0)
  constraints: 32 end point, 9 collinear, 2 coincident, 1 centre point, 1 concentric, 1 point on line, 4 other
extrude "Выдавливание2" add sketch "Эскиз3" along normal blind 5 contours A0 | A1 L4 L6 L8 L9 L12 L14 L17 L19 L23 L24 L28 L31 L32 L34 L1 L0 | L0 L1 A1 | A1 L6 L4 | L34 L32 A1 | A1 L9 L8 | L31 L28 A1 | A1 L14 L12 | L24 L23 A1 | A1 L19 L17
sketch "Эскиз4" plane through (0, 0, 5) normal (0, 0, -1) x (-1, 0, 0)
  line L0 (-9.7934, 11.7942) -> (-9.6836, 11.0043) projected
  arc A0 (-9.6836, 11.0043) -> (-9.1522, 12.2685) centre (-13.2452, 13.2452) ccw projected
  line L1 (-9.1522, 12.2685) -> (-9.7934, 11.7942) projected
  line L2 (-11.8305, 9.7784) -> (-12.3114, 9.1422) projected
  arc A1 (-12.3114, 9.1422) -> (-11.0417, 9.6604) centre (-13.2452, 13.2452) ccw projected
  line L3 (-11.0417, 9.6604) -> (-11.8305, 9.7784) projected
  line L4 (-14.6962, 9.7934) -> (-15.4862, 9.6836) projected
  arc A2 (-15.4862, 9.6836) -> (-14.222, 9.1522) centre (-13.2452, 13.2452) ccw projected
  line L5 (-14.222, 9.1522) -> (-14.6962, 9.7934) projected
  line L6 (-16.712, 11.8305) -> (-17.3483, 12.3114) projected
  arc A3 (-17.3483, 12.3114) -> (-16.8301, 11.0417) centre (-13.2452, 13.2452) ccw projected
  line L7 (-16.8301, 11.0417) -> (-16.712, 11.8305) projected
  line L8 (-17.3383, 14.222) -> (-16.697, 14.6962) projected
  line L9 (-16.697, 14.6962) -> (-16.8068, 15.4862) projected
  arc A4 (-16.8068, 15.4862) -> (-17.3383, 14.222) centre (-13.2452, 13.2452) ccw projected
  line L10 (-12.2685, 17.3383) -> (-11.7942, 16.697) projected
  line L11 (-11.7942, 16.697) -> (-11.0042, 16.8068) projected
  arc A5 (-11.0042, 16.8068) -> (-12.2685, 17.3383) centre (-13.2452, 13.2452) ccw projected
  line L12 (-15.4488, 16.8301) -> (-14.66, 16.712) projected
  line L13 (-14.66, 16.712) -> (-14.179, 17.3483) projected
  arc A6 (-14.179, 17.3483) -> (-15.4488, 16.8301) centre (-13.2452, 13.2452) ccw projected
  line L14 (-9.6604, 15.4488) -> (-9.7784, 14.66) projected
  line L15 (-9.7784, 14.66) -> (-9.1422, 14.179) projected
  arc A7 (-9.1422, 14.179) -> (-9.6604, 15.4488) centre (-13.2452, 13.2452) ccw projected
  point P0 (0, 0)
extrude "Выдавливание3" cut sketch "Эскиз4" against normal through all
sketch "Эскиз5" plane through (0, 0, 0) normal (0, 0, -1) x (-1, 0, 0)
  circle A0 centre (-13.2452, 13.2452) radius 1.5 projected
  circle A1 centre (-13.2452, 13.2452) radius 1.55
  line L0 (-14.7952, 12.1952) -> (-11.6952, 12.1952)
  line L1 (-11.6952, 12.1952) -> (-11.6952, 14.2952)
  line L2 (-11.6952, 14.2952) -> (-14.7952, 14.2952)
  line L3 (-14.7952, 14.2952) -> (-14.7952, 12.1952)
  line L4 (-14.7952, 12.1952) -> (-11.6952, 14.2952) construction
  line L5 (-11.6952, 12.1952) -> (-14.7952, 14.2952) construction
  point P0 (0, 0)
  point P1 (-14.3854, 12.1952)
  point P2 (-12.1051, 12.1952)
  dimension "d6" = 3.1
  dimension "d7" = 2.1
  constraints: 12 end point, 2 midpoint, 2 parallel, 1 centre point, 1 coincident, 1 horizontal, 1 perpendicular, 1 tangent
  measures "d6" diameter of A1
  measures "d7" distance of L0.end L1.end
extrude "Выдавливание4" cut sketch "Эскиз5" against normal through all contours A0 L0 L2 | A0 L2 A1 L0 | L2 A0 | A0 L2 A1 | A0 L0 A1 L2
sketch "Эскиз6" plane through (0, 0, 5) normal (0, 0, -1) x (-1, 0, 0)
  line L0 (-12.174, 12.1952) -> (-14.3165, 12.1952) projected
  arc A0 (-14.3165, 12.1952) -> (-12.174, 12.1952) centre (-13.2452, 13.2452) ccw projected
  point P0 (0, 0)
extrude "Выдавливание5" add sketch "Эскиз6" along normal up to surface (5 mm away)
fillet "Сопряжение1" radius 1 24 edges at (9.7194, 15.0544, 10) (9.4603, 14.4195, 10) (9.0373, 13.2232, 10) (9.4728, 12.0314, 10) (9.7385, 11.3992, 10) (10.2854, 10.2542, 10) (11.4361, 9.7194, 10) (12.0709, 9.4603, 10) (13.2673, 9.0373, 10) (14.4591, 9.4728, 10) (15.0912, 9.7385, 10) (16.2363, 10.2854, 10) (16.7711, 11.4361, 10) (17.0302, 12.0709, 10) (17.4531, 13.2673, 10) (17.0177, 14.4591, 10) (16.7519, 15.0912, 10) (16.2051, 16.2363, 10) (15.0544, 16.7711, 10) (14.4195, 17.0302, 10) (13.2232, 17.4531, 10) (12.0314, 17.0177, 10) (11.3992, 16.7519, 10) (10.2542, 16.2051, 10)
